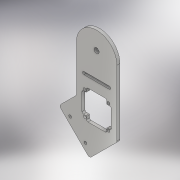
# Autodesk Inventor part: NEMA23MountPlatev2
Saved by Autodesk Inventor 2020.3 (Build 243373000, 373)
## iProperties
Created: 2021-09-06
Part Number: NEMA23MountPlatev2
Material: Aluminum 6061
Document SubType Name: Sheet Metal
Designer: justi
Density: 2.7 g/cm^3
Sheet Metal Rule: Default_mm
Appearance: Aluminum - Polished
Flat Pattern Width: 11.2175 cm
Flat Pattern Length: 22.3849 cm
Flat Pattern Area: 251.103 cm^2
Sheet Metal Width: 112.175 mm
Sheet Metal Length: 223.849 mm
Sheet Metal Area: 25110.314 mm^2
Author: justi
Autodesk Inventor part; units mm, degrees
ref_plane "YZ Plane" through (0, 0, 0) normal (1, 0, 0) x (0, 1, 0)
ref_plane "XZ Plane" through (0, 0, 0) normal (0, 1, 0) x (-1, 0, 0)
ref_plane "XY Plane" through (0, 0, 0) normal (0, 0, 1) x (1, 0, 0)
sketch "Sketch1" plane through (0, 0, 0) normal (0, 1, 0) x (-1, 0, 0)
  line L0 (40, 90) -> (-40, 90)
  line L1 (-40, 90) -> (-40, -81.7795)
  line L2 (40, -41.5685) -> (40, 90)
  line L3 (40, 90) -> (-40, -90) construction
  line L4 (-40, 90) -> (40, -90) construction
  line L5 (-0.0013, -90.0008) -> (-0.0013, 54.9992) construction
  circle A0 centre (-0.0013, 54.9992) radius 5.1
  line L6 (-0.0013, 54.9992) -> (-0.0013, -46.7008) construction
  line L7 (23.4987, -23.2008) -> (-23.5013, -23.2008) construction
  line L8 (-23.5013, -23.2008) -> (-23.5013, -70.2008) construction
  line L9 (-23.5013, -70.2008) -> (23.4987, -70.2008) construction
  line L10 (23.4987, -70.2008) -> (23.4987, -23.2008) construction
  line L11 (23.4987, -23.2008) -> (-23.5013, -70.2008) construction
  line L12 (-23.5013, -23.2008) -> (23.4987, -70.2008) construction
  circle A1 centre (23.4987, -23.2008) radius 2.75
  circle A2 centre (23.4987, -70.2008) radius 2.75
  circle A3 centre (-23.5013, -23.2008) radius 2.75
  circle A4 centre (-23.5013, -70.2008) radius 2.75
  line L13 (-0.0013, -90.0008) -> (-0.0013, -80) construction
  line L14 (19.9987, -17.7008) -> (-20.0013, -17.7008)
  line L15 (-20.0013, -17.7008) -> (-20.0013, -75.7008)
  line L16 (-20.0013, -75.7008) -> (19.9987, -75.7008)
  line L17 (19.9987, -75.7008) -> (19.9987, -17.7008)
  line L18 (19.9987, -17.7008) -> (-20.0013, -75.7008) construction
  line L19 (-20.0013, -17.7008) -> (19.9987, -75.7008) construction
  line L20 (-29.0013, -66.7008) -> (28.9987, -66.7008)
  line L21 (28.9987, -66.7008) -> (28.9987, -26.7008)
  line L22 (28.9987, -26.7008) -> (-29.0013, -26.7008)
  line L23 (-29.0013, -26.7008) -> (-29.0013, -66.7008)
  line L24 (-29.0013, -66.7008) -> (28.9987, -26.7008) construction
  line L25 (28.9987, -66.7008) -> (-29.0013, -26.7008) construction
  line L26 (-0.0013, 54.9992) -> (102.5291, -47.5313) construction
  line L27 (-0.0013, 54.9992) -> (144.9987, 54.9992) construction
  line L28 (28.2843, 83.2843) -> (-28.2843, 26.7157) construction
  line L29 (-28.2843, 26.7157) -> (74.2462, -75.8148) construction
  line L30 (74.2462, -75.8148) -> (130.8148, -19.2462) construction
  line L31 (130.8148, -19.2462) -> (28.2843, 83.2843) construction
  line L32 (28.2843, 83.2843) -> (74.2462, -75.8148) construction
  line L33 (-28.2843, 26.7157) -> (130.8148, -19.2462) construction
  line L34 (74.2462, -75.8148) -> (14.1407, -135.9202)
  line L35 (14.1407, -135.9202) -> (-0.0014, -121.7781)
  line L36 (-0.0014, -121.7781) -> (-31.7795, -90)
  line L37 (74.2462, -75.8148) -> (40, -41.5685)
  line L38 (-31.7795, -90) -> (-40, -81.7795)
  line L39 (44.1935, -105.8675) -> (37.1224, -98.7964)
  line L40 (37.1224, -98.7964) -> (52.1488, -83.7701) construction
  line L41 (37.1224, -98.7964) -> (22.096, -113.8228) construction
  circle A5 centre (52.1488, -83.7701) radius 2.75
  circle A6 centre (22.096, -113.8228) radius 2.75
  point P0 (0, 0)
  point P1 (51.2639, 3.7339)
  dimension "d0" = 80
  dimension "d1" = 180
  dimension "d2" = 145
  dimension "d3" = 10.2
  dimension "d4" = 101.7
  dimension "d5" = 47
  dimension "d6" = 47
  dimension "d7" = 5.5
  dimension "d8" = 5.5
  dimension "d9" = 5.5
  dimension "d10" = 5.5
  dimension "d12" = 40
  dimension "d13" = 58
  dimension "d14" = 58
  dimension "d15" = 40
  dimension "d27" = 45
  dimension "d28" = 145
  dimension "d29" = 80
  dimension "d30" = 145
  dimension "d31" = 85.002
  dimension "d32" = 20
  dimension "d33" = 10
  dimension "d35" = 21.2505
  dimension "d36" = 21.2505
  dimension "d37" = 5.5
  dimension "d38" = 5.5
  constraints: 84 end point, 10 midpoint, 10 parallel, 7 centre point, 7 coincident, 6 perpendicular, 5 horizontal, 5 point on line, 1 equal length, 1 vertical
  measures "d0" distance of L4.end L3.end
  measures "d1" distance of L3.end L0.end
  measures "d2" distance of L5.start L5.end
  measures "d3" diameter of A0
  measures "d4" distance of L6.start L6.end
  measures "d5" distance of L9.end L8.end
  measures "d6" distance of L8.end L7.end
  measures "d7" diameter of A1
  measures "d8" diameter of A2
  measures "d9" diameter of A3
  measures "d10" diameter of A4
  measures "d12" distance of L16.end L15.end
  measures "d13" distance of L15.end L14.end
  measures "d14" distance of L22.end L21.end
  measures "d15" distance of L21.end L20.end
  measures "d27" angle of L26 L27
  measures "d28" distance of L6.start L26.end
  measures "d29" distance of L30.end L29.end
  measures "d30" distance of L29.end L28.end
  measures "d31" distance of L29.end L34.end
  measures "d32" distance of L34.end L35.end
  measures "d33" distance of L39.start L39.end
  measures "d35" distance of L39.end L40.end
  measures "d36" distance of L39.end L41.end
  measures "d37" diameter of A5
  measures "d38" diameter of A6
extrude "Plate3" add sketch "Sketch1" along normal blind 6
fillet "Fillet6" radius 5 4 edges at (-40, 3, -41.5685) (-74.2462, 3, -75.8148) (-14.1407, 3, -135.9202) (40, 3, -81.7795)
fillet "Fillet7" radius 40 2 edges at (40, 3, 90) (-40, 3, 90)
sketch "Sketch2" plane through (0, 0, 0) normal (0, -1, 0) x (1, 0, 0)
  circle A0 centre (0.0013, 54.9992) radius 5.1 projected
  line L0 (0.0013, 54.9992) -> (0.0013, -46.7008) construction
  line L1 (0.0013, 4.1492) -> (55.0013, 4.1492) construction
  line L2 (0.0013, 4.1492) -> (-54.9987, 4.1492) construction
  line L3 (-24.9987, 4.1492) -> (25.0013, 4.1492) construction
  line L4 (-24.9987, 1.3992) -> (25.0013, 1.3992)
  line L5 (25.0013, 6.8992) -> (-24.9987, 6.8992)
  arc A1 (-24.9987, 6.8992) -> (-24.9987, 1.3992) centre (-24.9987, 4.1492) ccw
  arc A2 (25.0013, 1.3992) -> (25.0013, 6.8992) centre (25.0013, 4.1492) ccw
  point P0 (0, 0)
  dimension "d43" = 101.7
  dimension "d44" = 55
  dimension "d45" = 55
  dimension "d46" = 25
  dimension "d47" = 5.5
  constraints: 14 end point, 4 point on circle, 4 tangent, 2 centre point, 2 horizontal, 2 midpoint, 1 parallel, 1 point on line, 1 vertical
  measures "d43" distance of L0.start L0.end
  measures "d44" distance of L1.start L1.end
  measures "d45" distance of L1.start L2.end
  measures "d46" distance of L1.start L3.end
  measures "d47" diameter of A2
extrude "Extrusion1" cut sketch "Sketch2" against normal blind 10 contours A1 L5 A2 L4
fillet "Fillet9" radius 3 8 edges at (20.0013, 3, -17.7008) (29.0013, 3, -26.7008) (-28.9987, 3, -26.7008) (-19.9987, 3, -17.7008) (29.0013, 3, -66.7008) (20.0013, 3, -75.7008) (-28.9987, 3, -66.7008) (-19.9987, 3, -75.7008)
fillet "Fillet10" radius 1 4 edges at (-19.9987, 3, -26.7008) (20.0013, 3, -26.7008) (20.0013, 3, -66.7008) (-19.9987, 3, -66.7008)
ref_plane "Work Plane1" through (-24.9987, 0, 4.1492) normal (0, 0, 1) x (1, 0, 0)
equation "\"d39\" = Thickness"
equation "\"BendRadius\" = Thickness"
equation "\"BendReliefWidth\" = Thickness"
equation "\"BendReliefDepth\" = 0.5 * Thickness"
equation "\"CornerReliefSize\" = 4 * Thickness"
equation "\"MinimumRemnant\" = 2 * Thickness"
equation "\"TransitionRadius\" = BendRadius"
equation "\"JacobiRadiusSize\" = BendRadius"
equation "\"GapSize\" = Thickness"
equation "\"Thickness\" = 6"
body "Solid3"
